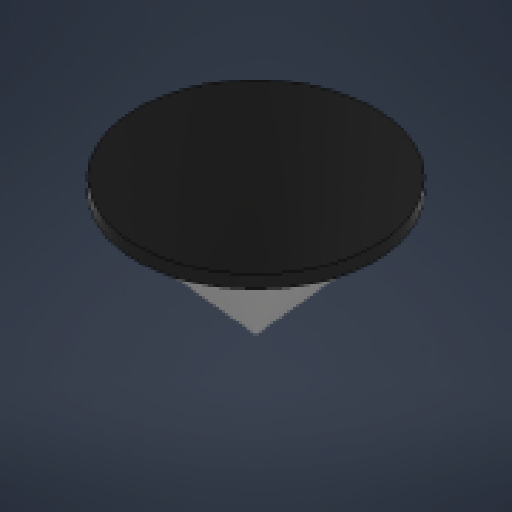
# Autodesk Inventor part: Camera_mirror
Saved by Autodesk Inventor 2024.2 (Build 282272000, 272)
## iProperties
Created: 2023-12-21
Part Number: Camera_mirror
Material: 一般
Document SubType Name: Modeling
Designer: Hanaoka
Density: 1 g/cm^3
Appearance: 既定
Author: Hanaoka
Autodesk Inventor part; units mm, degrees
ref_plane "YZ Plane" through (0, 0, 0) normal (1, 0, 0) x (0, 1, 0)
ref_plane "XZ Plane" through (0, 0, 0) normal (0, 1, 0) x (-1, 0, 0)
ref_plane "XY Plane" through (0, 0, 0) normal (0, 0, 1) x (1, 0, 0)
sketch "スケッチ1" plane through (0, 0, 0) normal (0, 0, 1) x (1, 0, 0)
  line L0 (-25, 28) -> (0, 0)
  line L1 (0, 0) -> (25, 28)
  line L2 (-25, 28) -> (25, 28)
  line L3 (0, 0) -> (0, 28) construction
  line L4 (-27, 31) -> (27, 31)
  line L5 (27, 31) -> (27, 28)
  line L6 (27, 28) -> (-27, 28)
  line L7 (-27, 28) -> (-27, 31)
  line L8 (0, -6.2) -> (0, 37.2) projected
  line L9 (0, 0) -> (0, 31)
  point P0 (25, 28)
  dimension "d0" = 50
  dimension "d1" = 28
  dimension "d2" = 54
  dimension "d3" = 3
  constraints: 18 end point, 2 horizontal, 2 midpoint, 2 parallel, 2 point on line, 1 coincident, 1 equal length, 1 perpendicular, 1 other
  measures "d0" distance of L0.start L1.end
  measures "d1" distance of L0.end L3.end
  measures "d2" distance of L4.start L4.end
  measures "d3" distance of L6.end L4.start
revolve "回転1" add sketch "スケッチ1" angle 360 about axis through (0, -10, 0) along (0, 1, 0) contours L8 L2 L1 | L8 L4 L5 L6 L2
